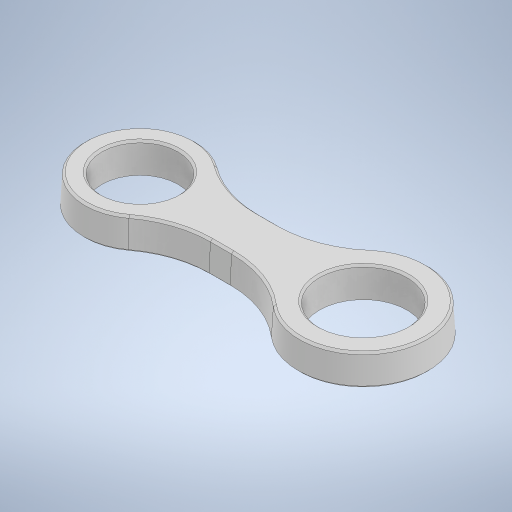
# Autodesk Inventor part: Connecting Rod Cast Image
Saved by Autodesk Inventor 2023 (Build 270158000, 158)
## iProperties
Created: 2022-10-29
Part Number: Connecting Rod Cast Image
Material: Generic
Document SubType Name: Modeling
Designer: tommy
Density: 1 g/cm^3
Appearance: Default
Author: tommy
Autodesk Inventor part; units mm, degrees
ref_plane "YZ Plane" through (0, 0, 0) normal (1, 0, 0) x (0, 1, 0)
ref_plane "XZ Plane" through (0, 0, 0) normal (0, 1, 0) x (-1, 0, 0)
ref_plane "XY Plane" through (0, 0, 0) normal (0, 0, 1) x (1, 0, 0)
sketch "Sketch1" plane through (0, 0, 0) normal (0, 1, 0) x (-1, 0, 0)
  circle A0 centre (-31.75, 0) radius 11.0744
  circle A1 centre (24.765, 0) radius 9.652
  line L0 (-16.51, -6.35) -> (11.9662, -6.35)
  circle A2 centre (24.765, 0) radius 14.2875
  circle A3 centre (-31.75, 0) radius 16.51
  line L1 (-16.51, 6.35) -> (11.9662, 6.35)
  point P0 (0, 0)
  dimension "d15" = 22.1488
  dimension "d17" = 12.7
  dimension "d18" = 33.02
  dimension "d19" = 19.304
  dimension "d20" = 28.575
  dimension "d21" = 56.515
  constraints: 4 centre point, 4 end point, 4 point on circle, 1 coincident, 1 concentric, 1 horizontal
  measures "d15" diameter of A0
  measures "d17" distance of L0.start L1.start
  measures "d18" diameter of A3
  measures "d19" diameter of A1
  measures "d20" diameter of A2
  measures "d21" distance of A1.centre A0.centre
extrude "Extrusion2" add sketch "Sketch1" along normal blind 7.62
fillet "Fillet3" radius 25.4 4 edges at (-11.9662, 3.81, 6.35) (-11.9662, 3.81, -6.35) (16.51, 3.81, -6.35) (16.51, 3.81, 6.35)
draft "FaceDraft2" angle 3 pull direction (0, 1, 0) faces at (41.7415, 5.08, -13.1435) (14.1702, 2.54, 8.307) (8.391, 2.54, -6.6666) (0.8295, 2.54, 6.35) (2.6114, 2.54, -6.35) (-2.7671, 2.54, 6.4149) (-4.5723, 2.54, -6.6093) (-18.1739, 5.08, 12.6764) fixed edges at (48.26, 0, 0) (13.2365, 0, 7.9391) (13.2365, 0, -7.9391) (1.7204, 0, 6.35) (1.7204, 0, -6.35) (-8.9847, 0, 7.6534) (-8.9847, 0, -7.6534) (-39.0525, 0, 0)
chamfer "Chamfer1" distance 0.508 angle 45 10 edges at (-38.6532, 7.62, 0) (-9.111, 7.62, 7.2746) (1.7204, 7.62, 5.9507) (13.3755, 7.62, 7.5647) (47.8607, 7.62, 0) (13.3755, 7.62, -7.5647) (1.7204, 7.62, -5.9507) (-9.111, 7.62, -7.2746) (42.8244, 7.62, 0) (-15.113, 7.62, 0)
chamfer "Chamfer2" distance 0.508 angle 45 8 edges at (13.2365, 0, 7.9391) (48.26, 0, 0) (13.2365, 0, -7.9391) (1.7204, 0, -6.35) (-8.9847, 0, -7.6534) (-39.0525, 0, 0) (-8.9847, 0, 7.6534) (1.7204, 0, 6.35)
body "Solid2"
